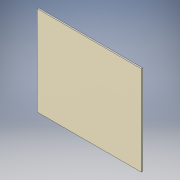
# Autodesk Inventor part: sheet
Saved by Autodesk Inventor 2019 (Build 230136000, 136)
## iProperties
Created: 2020-03-03
Part Number: sheet
Material: Generic
Document SubType Name: Modeling
Designer: Vinayak
Density: 1 g/cm^3
Appearance: Default
Author: Vinayak
Autodesk Inventor part; units mm, degrees
ref_plane "YZ Plane" through (0, 0, 0) normal (1, 0, 0) x (0, 1, 0)
ref_plane "XZ Plane" through (0, 0, 0) normal (0, 1, 0) x (-1, 0, 0)
ref_plane "XY Plane" through (0, 0, 0) normal (0, 0, 1) x (1, 0, 0)
sketch "Sketch1" plane through (0, 0, 0) normal (0, 0, 1) x (1, 0, 0)
  line L0 (0, 0) -> (-720, 0)
  line L1 (-720, 0) -> (-720, 620)
  line L2 (-720, 620) -> (0, 620)
  line L3 (0, 620) -> (0, 0)
  dimension "d6" = 720
  dimension "d7" = 620
  constraints: 8 end point, 2 parallel, 1 horizontal, 1 perpendicular
  measures "d6" distance of L1.end L2.end
  measures "d7" distance of L0.end L1.end
extrude "Extrusion1" add sketch "Sketch1" along normal blind 10
body "Solid1"
